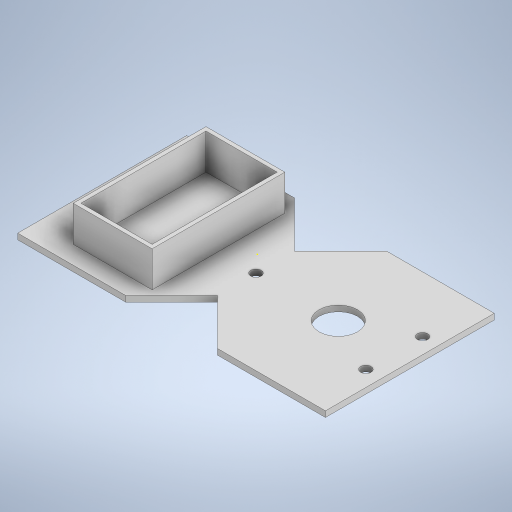
# Autodesk Inventor part: SCHOOL PROJECT TOP
Saved by Autodesk Inventor 2024 (Build 280153000, 153)
## iProperties
Created: 2025-05-09
Part Number: SCHOOL PROJECT TOP
Material: Generic
Document SubType Name: Modeling
Designer: arikm
Density: 1 g/cm^3
Appearance: Default
Author: arikm
Autodesk Inventor part; units mm, degrees
ref_plane "YZ Plane" through (0, 0, 0) normal (1, 0, 0) x (0, 1, 0)
ref_plane "XZ Plane" through (0, 0, 0) normal (0, 1, 0) x (-1, 0, 0)
ref_plane "XY Plane" through (0, 0, 0) normal (0, 0, 1) x (1, 0, 0)
sketch "Sketch1" plane through (0, 0, 0) normal (0, 1, 0) x (-1, 0, 0)
  line L0 (-88.0953, -35.095) -> (-78.6953, -35.095)
  line L1 (62.5047, 52.705) -> (71.9047, 52.705)
  line L2 (-88.0953, -35.095) -> (71.9047, -35.095)
  line L3 (71.9047, -35.095) -> (71.9047, 52.705)
  line L4 (71.9047, 52.705) -> (-88.0953, 52.705)
  line L5 (-88.0953, 52.705) -> (-88.0953, -35.095)
  circle A0 centre (-79.9551, -5.92) radius 2.7
  circle A1 centre (-79.9551, -5.92) radius 2.7
  circle A2 centre (-79.9551, 23.53) radius 2.7
  circle A3 centre (-79.9551, 23.53) radius 2.7
  circle A4 centre (-8.0953, 8.805) radius 2.7
  circle A5 centre (-8.0953, 8.805) radius 2.7
  circle A6 centre (63.7645, -5.92) radius 2.7
  circle A7 centre (63.7645, -5.92) radius 2.7
  circle A8 centre (63.7645, 23.53) radius 2.7
  circle A9 centre (63.7645, 23.53) radius 2.7
  line L6 (-88.0953, -35.095) -> (71.9047, -35.095)
  line L7 (71.9047, -35.095) -> (71.9047, 52.705)
  line L8 (71.9047, 52.705) -> (-88.0953, 52.705)
  line L9 (-88.0953, 52.705) -> (-88.0953, -35.095)
  point P0 (0, 0)
  point P1 (-83.0953, -33.095)
  constraints: 20 end point, 10 centre point, 5 coincident, 4 parallel, 2 horizontal, 2 perpendicular
extrude "Extrusion1" add sketch "Sketch1" along normal blind 3
sketch "Sketch2" plane through (0, 3, 0) normal (0, 1, 0) x (1, 0, 0)
  circle A0 centre (8.0953, -8.805) radius 2.7 projected
  line L0 (8.0953, -8.805) -> (8.0953, -52.705)
  line L1 (-71.9047, -52.705) -> (88.0953, -52.705) projected
  line L2 (8.0953, -8.805) -> (8.0953, 35.095)
  line L3 (88.0953, 35.095) -> (-71.9047, 35.095) projected
  line L4 (8.0953, -8.805) -> (-35.8047, -52.705)
  line L5 (8.0953, -8.805) -> (70.1793, -8.805) construction
  line L6 (8.0953, -8.805) -> (51.9953, -52.705)
  line L7 (8.0953, -8.805) -> (70.1793, -8.805) construction
  line L8 (8.0953, -8.805) -> (-18.3888, -8.805)
  line L9 (8.0953, -8.805) -> (-35.8047, 35.095)
  line L10 (8.0953, -8.805) -> (51.9953, 35.095)
  line L11 (-35.8047, -52.705) -> (51.9953, -52.705)
  line L12 (51.9953, -52.705) -> (51.9953, 35.095)
  line L13 (51.9953, 35.095) -> (-35.8047, 35.095)
  line L14 (-35.8047, 35.095) -> (-35.8047, -52.705)
  line L15 (8.0953, -8.805) -> (8.0953, -28.805)
  line L16 (8.0953, -28.805) -> (8.0953, 11.195)
  line L17 (8.0953, 11.195) -> (-15.8047, 35.095)
  line L18 (8.0953, -28.805) -> (-15.8047, -52.705)
  line L19 (8.0953, -28.805) -> (31.9953, -52.705)
  line L20 (8.0953, 11.195) -> (31.9953, 35.095)
  point P0 (0, 0)
  dimension "d2" = 135
  dimension "d3" = 45
  dimension "d4" = 20
  dimension "d5" = 40
  constraints: 38 end point, 8 point on line, 4 horizontal, 3 parallel, 2 equal length, 2 midpoint, 2 perpendicular, 2 symmetric about line
  measures "d2" angle of L4 L5
  measures "d3" angle of L6 L7
  measures "d4" distance of L0.start L15.end
  measures "d5" distance of L15.end L16.end
extrude "Extrusion2" cut sketch "Sketch2" against normal blind 3 contours L17 L3 L2 | L2 L3 L20 | L19 L1 L0 | L0 L1 L18
sketch "Sketch3" plane through (0, 3, 0) normal (0, 1, 0) x (1, 0, 0)
  line L0 (-71.9047, 35.095) -> (-71.9047, -52.705) projected
  line L1 (-71.9047, -8.805) -> (-34.7047, -8.805)
  circle A0 centre (-34.7047, -8.805) radius 10
  point P0 (0, 0)
  dimension "d8" = 37.2
  dimension "d9" = 20
  constraints: 2 end point, 1 centre point, 1 coincident, 1 horizontal, 1 midpoint
  measures "d8" distance of L1.start L1.end
  measures "d9" diameter of A0
extrude "Extrusion3" cut sketch "Sketch3" against normal blind 3
sketch "Sketch4" plane through (0, 3, 0) normal (0, 1, 0) x (1, 0, 0)
  point P0 (0, 0)
sketch "Sketch5" plane through (0, 3, 0) normal (0, 1, 0) x (1, 0, 0)
  line L0 (-71.9047, 35.095) -> (-71.9047, -52.705) projected
  line L1 (88.0953, -52.705) -> (88.0953, 35.095) projected
  line L2 (-71.9047, -52.705) -> (88.0953, -52.705)
  line L3 (8.0953, -52.705) -> (8.0953, 35.095)
  circle A0 centre (-34.7047, -8.805) radius 10 projected
  circle A1 centre (-34.7047, -8.805) radius 10
  circle A2 centre (50.8953, -8.805) radius 10
  point P0 (0, 0)
  constraints: 4 end point, 2 centre point, 1 coincident, 1 horizontal, 1 midpoint, 1 symmetric about line, 1 vertical, 1 other
extrude "Extrusion4" cut sketch "Sketch5" against normal blind 3 contours A2
sketch "Sketch6" plane through (0, 3, 0) normal (0, 1, 0) x (1, 0, 0)
  line L0 (-48.5025, 4.8798) -> (-18.5618, 4.8798)
  line L1 (-18.5618, 4.8798) -> (-18.5618, -20.2546)
  line L2 (-18.5618, -20.2546) -> (-48.5025, -20.2546)
  line L3 (-48.5025, -20.2546) -> (-48.5025, 4.8798)
  point P0 (0, 0)
  constraints: 8 end point, 2 parallel, 1 horizontal, 1 perpendicular
extrude "Extrusion5" add sketch "Sketch6" against normal up to surface (3 mm away)
sketch "Sketch7" plane through (0, 3, 0) normal (0, 1, 0) x (1, 0, 0)
  line L0 (-15.8047, 35.095) -> (-71.9047, 35.095) projected
  line L1 (-71.9047, 35.095) -> (8.0953, 35.095)
  line L2 (8.0953, 35.095) -> (8.0953, -52.705)
  line L3 (8.0953, -52.705) -> (-71.9047, -52.705)
  line L4 (-71.9047, -52.705) -> (-71.9047, 35.095)
  line L5 (-71.9047, -8.805) -> (8.0953, -8.805)
  line L6 (-31.9047, -8.805) -> (-52.4047, -8.805)
  line L7 (-52.4047, -8.805) -> (-11.4047, -8.805)
  line L8 (-52.4047, -8.805) -> (-11.4047, -8.805)
  line L9 (-11.4047, -8.805) -> (-11.4047, 25.695)
  line L10 (-11.4047, 25.695) -> (-52.4047, 25.695)
  line L11 (-52.4047, 25.695) -> (-52.4047, -8.805)
  line L12 (-52.4047, 25.695) -> (-11.4047, 25.695)
  line L13 (-11.4047, 25.695) -> (-11.4047, -43.305)
  line L14 (-11.4047, -43.305) -> (-52.4047, -43.305)
  line L15 (-52.4047, -43.305) -> (-52.4047, 25.695)
  line L16 (-31.9047, -8.805) -> (-31.9047, -5.9886)
  line L17 (-31.9047, -5.9886) -> (-50.3547, -5.9886)
  line L18 (-50.3547, -5.9886) -> (-13.4547, -5.9886)
  line L19 (-50.4047, 23.695) -> (-13.4047, 23.695)
  line L20 (-13.4047, 23.695) -> (-13.4047, -41.305)
  line L21 (-13.4047, -41.305) -> (-50.4047, -41.305)
  line L22 (-50.4047, -41.305) -> (-50.4047, 23.695)
  point P0 (0, 0)
  dimension "d16" = 20.5
  dimension "d17" = 41
  dimension "d18" = 34.5
  dimension "d19" = 69
  dimension "d20" = 18.45
  dimension "d21" = 36.9
  dimension "d22" = 2
  constraints: 44 end point, 8 parallel, 5 perpendicular, 4 point on line, 3 horizontal, 3 midpoint, 1 vertical, 3 other
  measures "d16" distance of L6.start L6.end
  measures "d17" distance of L6.end L7.end
  measures "d18" distance of L9.end L8.end
  measures "d19" distance of L12.end L13.end
  measures "d20" distance of L16.end L17.end
  measures "d21" distance of L17.end L18.end
  measures "d22" distance between parallel lines of L15 L22
extrude "Extrusion6" add sketch "Sketch7" along normal blind 18.5 contours L11 L10 L9 L5 L20 L19 L22 | L5 L22 L21 L20 L13 L14 L15
body "Solid1"
